Autodesk Inventor part; units mm, degrees
(part 11 of 11)
  line L90 (22.0183, 35.1028) -> (21.8234, 35.2977)
  arc A179 (26.1415, 34.4889) -> (26.1145, 34.5159) centre (26.128, 34.5024) ccw
  line L91 (25.9989, 34.3733) -> (25.9989, 34.2442)
  arc A180 (25.9799, 34.2442) -> (26.018, 34.2442) centre (25.9989, 34.2442) ccw
  arc A181 (26.018, 34.3733) -> (25.9799, 34.3733) centre (25.9989, 34.3733) ccw
  line L92 (25.9989, 34.2442) -> (26.5152, 34.2442)
  arc A182 (26.5152, 34.2252) -> (26.5152, 34.2633) centre (26.5152, 34.2442) ccw
  arc A183 (25.9989, 34.2633) -> (25.9989, 34.2252) centre (25.9989, 34.2442) ccw
  line L93 (24.4336, 33.9861) -> (24.9499, 33.9861)
  arc A184 (24.9499, 33.967) -> (24.9499, 34.0051) centre (24.9499, 33.9861) ccw
  arc A185 (24.4336, 34.0051) -> (24.4336, 33.967) centre (24.4336, 33.9861) ccw
  arc A186 (24.4471, 34.5159) -> (24.4201, 34.4889) centre (24.4336, 34.5024) ccw
  arc A187 (24.9364, 33.9726) -> (24.9634, 33.9996) centre (24.9499, 33.9861) ccw
  arc A188 (22.4081, 35.0774) -> (22.4081, 35.1282) centre (22.4081, 35.1028) ccw
  arc A189 (22.0183, 35.1282) -> (22.0183, 35.0774) centre (22.0183, 35.1028) ccw
  line L94 (22.4081, 35.1028) -> (22.0183, 35.1028)
  arc A190 (22.621, 35.2797) -> (22.5851, 35.3157) centre (22.603, 35.2977) ccw
  arc A191 (22.3902, 35.1208) -> (22.4261, 35.0848) centre (22.4081, 35.1028) ccw
  line L95 (22.603, 35.2977) -> (22.4081, 35.1028)
  line L96 (24.4336, 34.5024) -> (24.4336, 34.6315)
  arc A192 (24.4526, 34.6315) -> (24.4145, 34.6315) centre (24.4336, 34.6315) ccw
  arc A193 (24.4145, 34.5024) -> (24.4526, 34.5024) centre (24.4336, 34.5024) ccw
  arc A194 (22.6284, 36.0773) -> (22.5776, 36.0773) centre (22.603, 36.0773) ccw
  arc A195 (22.5776, 35.2977) -> (22.6284, 35.2977) centre (22.603, 35.2977) ccw
  line L97 (22.603, 36.0773) -> (22.603, 35.2977)
  arc A196 (22.4261, 36.2901) -> (22.3902, 36.2542) centre (22.4081, 36.2722) ccw
  arc A197 (22.5851, 36.0593) -> (22.621, 36.0953) centre (22.603, 36.0773) ccw
  line L98 (22.4081, 36.2722) -> (22.603, 36.0773)
  line L99 (24.4336, 34.6315) -> (24.5627, 34.7605)
  arc A198 (24.5761, 34.7471) -> (24.5492, 34.774) centre (24.5627, 34.7605) ccw
  arc A199 (24.4201, 34.645) -> (24.4471, 34.618) centre (24.4336, 34.6315) ccw
  line L100 (24.5627, 34.7605) -> (24.8208, 34.7605)
  arc A200 (24.8208, 34.7415) -> (24.8208, 34.7796) centre (24.8208, 34.7605) ccw
  arc A201 (24.5627, 34.7796) -> (24.5627, 34.7415) centre (24.5627, 34.7605) ccw
  arc A202 (22.0183, 36.2976) -> (22.0183, 36.2468) centre (22.0183, 36.2722) ccw
  arc A203 (22.4081, 36.2468) -> (22.4081, 36.2976) centre (22.4081, 36.2722) ccw
  line L101 (22.0183, 36.2722) -> (22.4081, 36.2722)
  arc A204 (21.8055, 36.0953) -> (21.8414, 36.0593) centre (21.8234, 36.0773) ccw
  arc A205 (22.0363, 36.2542) -> (22.0004, 36.2902) centre (22.0183, 36.2722) ccw
  line L102 (21.8234, 36.0773) -> (22.0183, 36.2722)
  arc A206 (22.9674, 35.2977) -> (23.0182, 35.2977) centre (22.9928, 35.2977) ccw
  arc A207 (23.0182, 36.2722) -> (22.9674, 36.2722) centre (22.9928, 36.2722) ccw
  line L103 (22.9928, 35.2977) -> (22.9928, 36.2722)
  arc A208 (23.1698, 35.0848) -> (23.2057, 35.1208) centre (23.1877, 35.1028) ccw
  arc A209 (23.0108, 35.3157) -> (22.9749, 35.2797) centre (22.9928, 35.2977) ccw
  line L104 (23.1877, 35.1028) -> (22.9928, 35.2977)
  line L105 (24.8208, 34.7605) -> (24.9499, 34.6315)
  arc A210 (24.9364, 34.618) -> (24.9634, 34.645) centre (24.9499, 34.6315) ccw
  arc A211 (24.8343, 34.774) -> (24.8073, 34.7471) centre (24.8208, 34.7605) ccw
  line L106 (24.1672, 34.1152) -> (24.1672, 34.6315)
  arc A212 (24.1863, 34.6315) -> (24.1482, 34.6315) centre (24.1672, 34.6315) ccw
  arc A213 (24.1482, 34.1152) -> (24.1863, 34.1152) centre (24.1672, 34.1152) ccw
  line L107 (24.1672, 34.6315) -> (24.0381, 34.7606)
  arc A214 (24.0516, 34.774) -> (24.0247, 34.7471) centre (24.0381, 34.7606) ccw
  arc A215 (24.1537, 34.618) -> (24.1807, 34.645) centre (24.1672, 34.6315) ccw
  line L108 (24.0381, 34.7606) -> (23.78, 34.7606)
  arc A216 (23.78, 34.7796) -> (23.78, 34.7415) centre (23.78, 34.7606) ccw
  arc A217 (24.0381, 34.7415) -> (24.0381, 34.7796) centre (24.0381, 34.7606) ccw
  line L109 (23.78, 34.7606) -> (23.6509, 34.6315)
  arc A218 (23.6374, 34.645) -> (23.6644, 34.618) centre (23.6509, 34.6315) ccw
  arc A219 (23.7935, 34.7471) -> (23.7665, 34.774) centre (23.78, 34.7606) ccw
  line L110 (23.6509, 34.6315) -> (23.6509, 34.1152)
  arc A220 (23.6319, 34.1152) -> (23.67, 34.1152) centre (23.6509, 34.1152) ccw
  arc A221 (23.67, 34.6315) -> (23.6319, 34.6315) centre (23.6509, 34.6315) ccw
  arc A222 (23.5775, 35.0774) -> (23.5775, 35.1282) centre (23.5775, 35.1028) ccw
  arc A223 (23.1877, 35.1282) -> (23.1877, 35.0774) centre (23.1877, 35.1028) ccw
  line L111 (23.5775, 35.1028) -> (23.1877, 35.1028)
  arc A224 (23.7904, 35.2797) -> (23.7545, 35.3157) centre (23.7724, 35.2977) ccw
  arc A225 (23.5596, 35.1208) -> (23.5955, 35.0848) centre (23.5775, 35.1028) ccw
  line L112 (23.7724, 35.2977) -> (23.5775, 35.1028)
  arc A226 (23.7978, 36.2722) -> (23.747, 36.2722) centre (23.7724, 36.2722) ccw
  arc A227 (23.747, 35.2977) -> (23.7978, 35.2977) centre (23.7724, 35.2977) ccw
  line L113 (23.7724, 36.2722) -> (23.7724, 35.2977)
  arc A228 (24.1442, 36.0953) -> (24.1802, 36.0593) centre (24.1622, 36.0773) ccw
  arc A229 (24.3751, 36.2542) -> (24.3392, 36.2901) centre (24.3571, 36.2722) ccw
  line L114 (24.1622, 36.0773) -> (24.3571, 36.2722)
  arc A230 (24.1368, 35.2977) -> (24.1876, 35.2977) centre (24.1622, 35.2977) ccw
  arc A231 (24.1876, 36.0773) -> (24.1368, 36.0773) centre (24.1622, 36.0773) ccw
  line L115 (24.1622, 35.2977) -> (24.1622, 36.0773)
  arc A232 (24.3392, 35.0849) -> (24.3751, 35.1208) centre (24.3571, 35.1028) ccw
  arc A233 (24.1802, 35.3157) -> (24.1442, 35.2797) centre (24.1622, 35.2977) ccw
  line L116 (24.3571, 35.1028) -> (24.1622, 35.2977)
  arc A234 (24.7469, 35.0774) -> (24.7469, 35.1282) centre (24.7469, 35.1028) ccw
  arc A235 (24.3571, 35.1282) -> (24.3571, 35.0774) centre (24.3571, 35.1028) ccw
  line L117 (24.7469, 35.1028) -> (24.3571, 35.1028)
  arc A236 (24.9598, 35.2797) -> (24.9239, 35.3157) centre (24.9418, 35.2977) ccw
  arc A237 (24.729, 35.1208) -> (24.7649, 35.0848) centre (24.7469, 35.1028) ccw
  line L118 (24.9418, 35.2977) -> (24.7469, 35.1028)
  arc A238 (24.9672, 36.0773) -> (24.9164, 36.0773) centre (24.9418, 36.0773) ccw
  arc A239 (24.9164, 35.2977) -> (24.9672, 35.2977) centre (24.9418, 35.2977) ccw
  line L119 (24.9418, 36.0773) -> (24.9418, 35.2977)
  arc A240 (24.7649, 36.2901) -> (24.729, 36.2542) centre (24.7469, 36.2722) ccw
  arc A241 (24.9238, 36.0593) -> (24.9598, 36.0952) centre (24.9418, 36.0773) ccw
  line L120 (24.7469, 36.2722) -> (24.9418, 36.0773)
  arc A242 (24.3571, 36.2976) -> (24.3571, 36.2468) centre (24.3571, 36.2722) ccw
  arc A243 (24.7469, 36.2468) -> (24.7469, 36.2976) centre (24.7469, 36.2722) ccw
  line L121 (24.3571, 36.2722) -> (24.7469, 36.2722)
  line L122 (23.6509, 34.1152) -> (23.78, 33.9861)
  arc A244 (23.7665, 33.9726) -> (23.7935, 33.9996) centre (23.78, 33.9861) ccw
  arc A245 (23.6644, 34.1286) -> (23.6374, 34.1017) centre (23.6509, 34.1152) ccw
  line L123 (23.78, 33.9861) -> (24.0381, 33.9861)
  arc A246 (24.0381, 33.967) -> (24.0381, 34.0051) centre (24.0381, 33.9861) ccw
  arc A247 (23.78, 34.0051) -> (23.78, 33.967) centre (23.78, 33.9861) ccw
  arc A248 (26.1112, 36.2468) -> (26.1112, 36.2976) centre (26.1112, 36.2722) ccw
  arc A249 (25.3316, 36.2976) -> (25.3316, 36.2468) centre (25.3316, 36.2722) ccw
  line L124 (26.1112, 36.2722) -> (25.3316, 36.2722)
  arc A250 (25.696, 35.1028) -> (25.7468, 35.1028) centre (25.7214, 35.1028) ccw
  arc A251 (25.7468, 36.2722) -> (25.696, 36.2722) centre (25.7214, 36.2722) ccw
  line L125 (25.7214, 35.1028) -> (25.7214, 36.2722)
  line L126 (24.0381, 33.9861) -> (24.1672, 34.1152)
  arc A252 (24.1807, 34.1017) -> (24.1538, 34.1286) centre (24.1672, 34.1152) ccw
  arc A253 (24.0247, 33.9996) -> (24.0516, 33.9726) centre (24.0381, 33.9861) ccw
  line L127 (24.1672, 34.1152) -> (23.6509, 34.6315)
  arc A254 (23.6644, 34.645) -> (23.6374, 34.618) centre (23.6509, 34.6315) ccw
  arc A255 (24.1537, 34.1017) -> (24.1807, 34.1286) centre (24.1672, 34.1152) ccw
  line L128 (23.3846, 34.5024) -> (23.1264, 34.7606)
  arc A256 (23.1399, 34.774) -> (23.1129, 34.7471) centre (23.1264, 34.7606) ccw
  arc A257 (23.3711, 34.4889) -> (23.398, 34.5159) centre (23.3846, 34.5024) ccw
  line L129 (23.1264, 34.7606) -> (23.1264, 33.9861)
  arc A258 (23.1073, 33.9861) -> (23.1454, 33.9861) centre (23.1264, 33.9861) ccw
  arc A259 (23.1454, 34.7606) -> (23.1073, 34.7606) centre (23.1264, 34.7606) ccw
  arc A260 (27.645, 35.1028) -> (27.6958, 35.1028) centre (27.6704, 35.1028) ccw
  arc A261 (27.6958, 36.2722) -> (27.645, 36.2722) centre (27.6704, 36.2722) ccw
  line L130 (27.6704, 35.1028) -> (27.6704, 36.2722)
  arc A262 (28.4711, 36.2581) -> (28.4289, 36.2863) centre (28.45, 36.2722) ccw
  arc A263 (27.6493, 35.1169) -> (27.6915, 35.0887) centre (27.6704, 35.1028) ccw
  line L131 (28.45, 36.2722) -> (27.6704, 35.1028)
  arc A264 (28.4246, 35.1028) -> (28.4754, 35.1028) centre (28.45, 35.1028) ccw
  arc A265 (28.4754, 36.2722) -> (28.4246, 36.2722) centre (28.45, 36.2722) ccw
  line L132 (28.45, 35.1028) -> (28.45, 36.2722)
  constraints: 676 point on circle, 266 centre point, 266 end point, 93 point on line, 10 midpoint
sketch "44" plane through (0, 0, 0) normal (0, 0, 1) x (1, 0, 0)
  circle A0 centre (33.528, 17.78) radius 0.1651
  circle A1 centre (31.75, 33.528) radius 0.1651
  circle A2 centre (10.668, 9.398) radius 0.1651
  circle A3 centre (17.78, 13.208) radius 0.1651
  circle A4 centre (34.29, 16.256) radius 0.1651
  circle A5 centre (14.732, 16.51) radius 0.1651
  circle A6 centre (27.432, 10.668) radius 0.1651
  circle A7 centre (20.828, 15.494) radius 0.1651
  circle A8 centre (35.56, 28.194) radius 0.1651
  circle A9 centre (4.064, 31.242) radius 0.1651
  circle A10 centre (9.398, 20.32) radius 0.1651
  circle A11 centre (32.512, 32.766) radius 0.1651
  circle A12 centre (12.2461, 17.8305) radius 0.1651
  circle A13 centre (11.176, 20.32) radius 0.1651
  circle A14 centre (14.986, 22.098) radius 0.1651
  circle A15 centre (12.954, 26.67) radius 0.1651
  circle A16 centre (26.162, 27.432) radius 0.1651
  circle A17 centre (9.398, 26.162) radius 0.1651
  circle A18 centre (5.588, 34.036) radius 0.1651
  circle A19 centre (17.018, 22.352) radius 0.1651
  circle A20 centre (16.002, 15.494) radius 0.1651
  circle A21 centre (30.988, 34.29) radius 0.1651
  circle A22 centre (15.494, 30.226) radius 0.1651
  constraints: 23 centre point, 22 equal radius
extrude "Extrusion1" add sketch "20" along normal blind 0.6096 contours L7 A27 A1 A25 A23 A26 L6 A37 L5 A20 A22 A18 A16 A19 L4 A34 L3 A13 A15 A11 A9 A12 L2 A31 L1 A6 A8 A4 L0 A28 | L7 A25 A1 A27 | A25 L6 A26 A23 | A8 A6 L1 A4 | L5 A18 A22 A20 | A18 L4 A19 A16 | A12 A9 A11 L2 | A15 A13 L3 A11 picked at (0.0369, 31.6948) picked at (5.1452, 36.817) picked at (32.7008, 36.817) picked at (36.817, 32.7008) picked at (31.6948, 0.0369) picked at (36.817, 5.1452)
body "Solid1"
